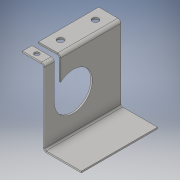
# Autodesk Inventor part: Tape Measure Dispenser Part 2
Saved by Autodesk Inventor 2016 (Build 200138000, 138)
## iProperties
Created: 2016-02-03
Part Number: Tape Measure Dispenser Part 2
Material: Generic
Document SubType Name: Sheet Metal
Designer: GEH-Magnet School 1
Density: 1 g/cm^3
Sheet Metal Rule: Default
Appearance: Default
Author: GEH-Magnet School 1
Autodesk Inventor part; units mm, degrees
note: some values were not read from the file. Chosen so that the rebuilt part matches the saved one: flange form of "Plate2".
ref_plane "YZ Plane" through (0, 0, 0) normal (1, 0, 0) x (0, 1, 0)
ref_plane "XZ Plane" through (0, 0, 0) normal (0, 1, 0) x (-1, 0, 0)
ref_plane "XY Plane" through (0, 0, 0) normal (0, 0, 1) x (1, 0, 0)
sketch "Sketch1" plane through (0, 0, 0) normal (0, 1, 0) x (-1, 0, 0)
  line L0 (-9.7302, 52.2849) -> (-85.9302, 52.2849)
  line L1 (-85.9302, 52.2849) -> (-85.9302, -100.1151)
  line L2 (-85.9302, -100.1151) -> (-9.7302, -100.1151)
  line L3 (-9.7302, -100.1151) -> (-9.7302, 52.2849)
  point P0 (0, 0)
  dimension "d0" = 152.4
  dimension "d1" = 76.2
  measures "d0" distance of L0.end L1.end
  measures "d1" distance of L0.start L0.end
extrude "Plate1" add sketch "Sketch1" along normal blind 3.048
sketch "Sketch2" plane through (12.7782, 0, 52.2849) normal (-1, 0, 0) x (0, -1, 0)
  line L0 (0, -152.4) -> (0, 0)
  line L1 (0, 0) -> (-152.4, 0)
  line L2 (-152.4, 0) -> (-152.4, -152.4)
  line L3 (-152.4, -152.4) -> (0, -152.4)
  constraints: 6 end point, 1 horizontal, 1 perpendicular, 1 vertical
edge flange "Flange1" height 152.4 angle 90 thickness 3.048 bend radius 3.048 thickness toward (-1, 0, 0) relief tear relief width 3.048 relief depth 1.524 edges at (9.7302, 3.048, -23.9151) wall of the first edge with corners at (12.7782, 0, -100.1151) (12.7782, 0, 52.2849) (12.7782, 152.4, 52.2849) (12.7782, 152.4, -100.1151)
bend "Bend1"
corner "Corner1"
sketch "Sketch5" plane through (12.7782, 152.4, 52.2849) normal (1, 0, 0) x (0, 0, -1)
  circle A0 centre (57.15, -76.2) radius 38.1
  line L0 (0, -152.4) -> (152.4, -152.4) projected
  line L1 (152.4, 0) -> (152.4, -146.304) projected
  point P0 (52.2849, -152.4)
  dimension "d23" = 76.2
  dimension "d24" = 76.2
  dimension "d25" = 95.25
  constraints: 1 centre point
  measures "d23" diameter of A0
  measures "d24" distance from line of L0 A0.centre
  measures "d25" distance from line of L1 A0.centre
extrude "Cut1" cut sketch "Sketch5" against normal blind 3.048
sketch "Sketch6" plane through (12.7782, 152.4, 52.2849) normal (1, 0, 0) x (0, 0, -1)
  circle A0 centre (57.15, -76.2) radius 38.1 projected
  line L0 (19.05, -76.2) -> (19.05, 0)
  line L1 (152.4, 0) -> (0, 0) projected
  line L2 (19.05, 0) -> (31.75, 0)
  line L3 (31.75, 0) -> (31.75, -47.8019)
  arc A1 (31.75, -47.8019) -> (19.05, -76.2) centre (57.15, -76.2) ccw
  point P0 (52.2849, -152.4)
  dimension "d47" = 12.7
  constraints: 6 end point, 4 point on circle, 2 point on line, 2 tangent, 1 centre point, 1 concentric, 1 perpendicular, 1 vertical
  measures "d47" distance of L2.end L0.end
extrude "Cut2" cut sketch "Sketch6" against normal blind 3.048 contours A0 L0 L1 L3
sketch "Sketch7" plane through (12.7782, 149.352, 33.2349) normal (0, 1, 0) x (-1, 0, 0)
  line L0 (0, 19.05) -> (0, 0)
  line L1 (0, 0) -> (44.45, 0)
  line L2 (44.45, 0) -> (44.45, 19.05)
  line L3 (44.45, 19.05) -> (0, 19.05)
  constraints: 6 end point, 1 horizontal, 1 perpendicular, 1 vertical
edge flange "Flange3" height 44.45 angle 90 thickness 3.048 bend radius 3.048 thickness toward (0, 1, 0) relief tear relief width 3.048 relief depth 1.524 corner gap 3.048 corner form 0 edges at (9.7302, 152.4, 42.7599) (9.7302, 152.4, -39.7901) wall of the first edge with corners at (12.7782, 149.352, 52.2849) (12.7782, 149.352, 33.2349) (-31.6718, 149.352, 33.2349) (-31.6718, 149.352, 52.2849)
bend "Bend3"
corner "Corner3"
sketch "Sketch8" plane through (-31.6718, 152.4, 20.5349) normal (0, 1, 0) x (1, 0, 0)
  circle A0 centre (19.05, 95.25) radius 6.35
  circle A1 centre (19.05, 25.4) radius 6.35
  line L0 (38.354, 0) -> (0, 0) projected
  line L1 (0, 0) -> (0, 120.65) projected
  point P0 (31.6718, 20.5349)
  dimension "d40" = 12.7
  dimension "d41" = 69.85
  dimension "d42" = 25.4
  dimension "d43" = 19.05
  dimension "d44" = 19.05
  constraints: 2 centre point
  measures "d40" diameter of A0
  measures "d41" distance of A1.centre A0.centre
  measures "d42" distance from line of A1.centre L0
  measures "d43" distance from line of L1 A0.centre
  measures "d44" distance from line of L1 A1.centre
extrude "Cut3" cut sketch "Sketch8" against normal blind 3.048
sketch "Sketch9" plane through (-31.6718, 152.4, 52.2849) normal (0, 1, 0) x (1, 0, 0)
  circle A0 centre (19.05, 9.525) radius 4.7625
  line L0 (38.354, 0) -> (0, 0) projected
  line L1 (0, 0) -> (0, 19.05) projected
  point P0 (31.6718, 52.2849)
  dimension "d48" = 9.525
  dimension "d49" = 9.525
  dimension "d50" = 19.05
  constraints: 1 centre point
  measures "d48" diameter of A0
  measures "d49" distance from line of L0 A0.centre
  measures "d50" distance from line of L1 A0.centre
extrude "Cut4" cut sketch "Sketch9" against normal blind 3.048
sketch "Sketch10" plane through (-31.6718, 149.352, 20.5349) normal (0, 0, 1) x (1, 0, 0)
  point P0 (31.6718, -149.352)
sketch "Sketch11" plane through (0, 3.048, 0) normal (0, 1, 0) x (1, 0, 0)
  circle A0 centre (66.8802, -42.7599) radius 3.175
  circle A1 centre (28.7802, -42.7599) radius 3.175
  line L0 (85.9302, -52.2849) -> (15.8262, -52.2849) projected
  line L1 (85.9302, 100.1151) -> (85.9302, -52.2849) projected
  circle A2 centre (66.8802, 90.5901) radius 3.175
  circle A3 centre (28.7802, 90.5901) radius 3.175
  line L2 (15.8262, 100.1151) -> (85.9302, 100.1151) projected
  point P0 (0, 0)
  dimension "d53" = 6.35
  dimension "d54" = 6.35
  dimension "d55" = 9.525
  dimension "d56" = 9.525
  dimension "d57" = 38.1
  dimension "d58" = 19.05
  dimension "d59" = 6.35
  dimension "d60" = 6.35
  dimension "d63" = 38.1
  dimension "d65" = 9.525
  dimension "d66" = 9.525
  dimension "d67" = 19.05
  constraints: 4 centre point
  measures "d53" diameter of A0
  measures "d54" diameter of A1
  measures "d55" distance from line of L0 A1.centre
  measures "d56" distance from line of L0 A0.centre
  measures "d57" distance of A0.centre A1.centre
  measures "d58" distance from line of L1 A0.centre
  measures "d59" diameter of A2
  measures "d60" diameter of A3
  measures "d63" distance of A2.centre A3.centre
  measures "d65" distance from line of L2 A2.centre
  measures "d66" distance from line of L2 A3.centre
  measures "d67" distance from line of L1 A2.centre
extrude "Cut5" cut sketch "Sketch11" against normal blind 3.048
equation "\"d26\" = Thickness"
equation "\"d28\" = Thickness"
equation "\"d45\" = Thickness"
equation "\"d51\" = Thickness"
equation "\"d68\" = Thickness"
equation "\"d3\" = BendReliefWidth"
equation "\"d4\" = BendReliefDepth"
equation "\"d5\" = MinimumRemnant"
equation "\"d6\" = BendRadius"
equation "\"d9\" = BendRadius"
equation "\"d10\" = CornerReliefSize"
equation "\"d11\" = GapSize"
equation "\"d12\" = JacobiRadiusSize"
equation "\"d30\" = BendReliefWidth"
equation "\"d31\" = BendReliefDepth"
equation "\"d32\" = MinimumRemnant"
equation "\"d33\" = BendRadius"
equation "\"d36\" = BendRadius"
equation "\"d37\" = CornerReliefSize"
equation "\"d38\" = GapSize"
equation "\"d39\" = JacobiRadiusSize"
equation "\"BendRadius\" = Thickness"
equation "\"BendReliefWidth\" = Thickness"
equation "\"BendReliefDepth\" = 0.5 * Thickness"
equation "\"CornerReliefSize\" = 4 * Thickness"
equation "\"MinimumRemnant\" = 2 * Thickness"
equation "\"TransitionRadius\" = BendRadius"
equation "\"JacobiRadiusSize\" = BendRadius"
equation "\"GapSize\" = Thickness"
equation "\"d2\" = BendRadius"
equation "\"Thickness\" = 3.048"
body "Solid1"
